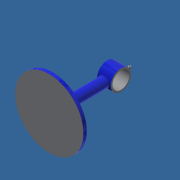
# Autodesk Inventor part: Feet
Saved by Autodesk Inventor 2018 (Build 220112000, 112)
## iProperties
Created: 2022-02-21
Part Number: Feet
Material: Generic
Document SubType Name: Modeling
Designer: Nathann
Density: 1 g/cm^3
Appearance: Default
Author: Nathann
Autodesk Inventor part; units mm, degrees
ref_plane "YZ Plane" through (0, 0, 0) normal (1, 0, 0) x (0, 1, 0)
ref_plane "XZ Plane" through (0, 0, 0) normal (0, 1, 0) x (-1, 0, 0)
ref_plane "XY Plane" through (0, 0, 0) normal (0, 0, 1) x (1, 0, 0)
sketch "Sketch1" plane through (0, 0, 0) normal (0, 1, 0) x (-1, 0, 0)
  circle A0 centre (0, 0) radius 100
  dimension "d0" = 200
  constraints: 1 centre point, 1 coincident
  measures "d0" diameter of A0
extrude "Extrusion1" add sketch "Sketch1" along normal blind 10
sketch "Sketch2" plane through (0, 10, 0) normal (0, 1, 0) x (1, 0, 0)
  circle A0 centre (0, 0) radius 15
  dimension "d5" = 30
  constraints: 1 centre point, 1 coincident
  measures "d5" diameter of A0
extrude "Extrusion2" add sketch "Sketch2" along normal blind 150
fillet "Fillet1" radius 20 1 edges at (-15, 10, 0)
sketch "Sketch3" plane through (0, 0, 0) normal (1, 0, 0) x (0, 1, 0)
  circle A0 centre (190, 0) radius 30
  line L0 (160, -15) -> (160, 15) projected
  circle A1 centre (190, 0) radius 25
  point P0 (0, 0)
  dimension "d7" = 50
  dimension "d8" = 60
  constraints: 2 centre point, 1 coincident, 1 tangent
  measures "d7" diameter of A1
  measures "d8" diameter of A0
extrude "Extrusion3" add sketch "Sketch3" along normal mid plane 40
sketch "Sketch4" plane through (0, 0, 0) normal (0, 0, 1) x (1, 0, 0)
  line L0 (-20, 220) -> (20, 220) projected
  line L1 (-1.546, 220) -> (1.9488, 220)
  line L2 (1.9488, 220) -> (1.9488, 232.6856)
  line L3 (-1.546, 232.4383) -> (-1.546, 220)
  circle A0 centre (0, 235.4083) radius 3.3482
  circle A1 centre (0, 235.4083) radius 1.5
  point P0 (0, 0)
  dimension "d11" = 3
  constraints: 6 end point, 2 centre point, 2 point on circle, 1 coincident, 1 horizontal, 1 parallel, 1 perpendicular, 1 point on line
  measures "d11" diameter of A1
extrude "Extrusion4" add sketch "Sketch4" along normal mid plane 5
body "Solid1"
